Autodesk Inventor part; units mm, degrees
(part 5 of 5)
  arc A545 (140.0996, 136.9129) -> (139.9695, 135.8932) centre (152.2699, 134.8417) ccw projected
  arc A546 (140.8649, 137.1046) -> (140.0996, 136.9129) centre (148.5, 105) ccw projected
  arc A547 (141.4603, 136.2666) -> (140.8649, 137.1046) centre (131.108, 129.5409) ccw projected
  arc A548 (141.8604, 135.5943) -> (141.4603, 136.2666) centre (133.1536, 130.8684) ccw projected
  arc A549 (141.9516, 135.4211) -> (141.8604, 135.5943) centre (135.198, 131.976) ccw projected
  arc A550 (141.9516, 135.4211) -> (142.4946, 135.1579) centre (142.397, 135.6483) ccw projected
  arc A551 (142.5073, 135.1604) -> (142.4946, 135.1579) centre (148.5, 105) ccw projected
  arc A552 (142.5073, 135.1604) -> (142.9083, 135.6114) centre (142.4099, 135.6508) ccw projected
  arc A553 (142.9263, 135.8063) -> (142.9083, 135.6114) centre (150.4662, 135.013) ccw projected
  arc A554 (143.0386, 136.5805) -> (142.9263, 135.8063) centre (152.7789, 134.7721) ccw projected
  arc A555 (143.2681, 137.5826) -> (143.0386, 136.5805) centre (155.1767, 134.3285) ccw projected
  arc A556 (144.0484, 137.6984) -> (143.2681, 137.5826) centre (148.5, 105) ccw projected
  arc A557 (144.5589, 136.8061) -> (144.0484, 137.6984) centre (133.5972, 131.1274) ccw projected
  arc A558 (144.8911, 136.0978) -> (144.5589, 136.8061) centre (135.763, 132.248) ccw projected
  arc A559 (144.9649, 135.9164) -> (144.8911, 136.0978) centre (137.9061, 133.1499) ccw projected
  arc A560 (144.9649, 135.9164) -> (145.4796, 135.6013) centre (145.4304, 136.0989) ccw projected
  arc A561 (145.4924, 135.6026) -> (145.4796, 135.6013) centre (148.5, 105) ccw projected
  arc A562 (145.4924, 135.6026) -> (145.9357, 136.012) centre (145.4435, 136.1002) ccw projected
  arc A563 (145.9727, 136.2043) -> (145.9357, 136.012) centre (153.3985, 134.6758) ccw projected
  arc A564 (146.1603, 136.9638) -> (145.9727, 136.2043) centre (155.6764, 134.2093) ccw projected
  arc A565 (146.4869, 137.9385) -> (146.1603, 136.9638) centre (158.0193, 133.5328) ccw projected
  arc A566 (147.2749, 137.9773) -> (146.4869, 137.9385) centre (148.5, 105) ccw projected
  arc A567 (147.6954, 137.0392) -> (147.2749, 137.9773) centre (136.2299, 132.4624) ccw projected
  arc A568 (147.9566, 136.3017) -> (147.6954, 137.0392) centre (138.4951, 133.3653) ccw projected
  arc A569 (148.0123, 136.1141) -> (147.9566, 136.3017) centre (140.7163, 134.0527) ccw projected
  arc A570 (148.0123, 136.1141) -> (148.4935, 135.75) centre (148.4934, 136.25) ccw projected
  arc A571 (148.5065, 135.75) -> (148.4935, 135.75) centre (148.5, 105) ccw projected
  arc A572 (148.5065, 135.75) -> (148.9877, 136.1141) centre (148.5066, 136.25) ccw projected
  arc A573 (149.0434, 136.3017) -> (148.9877, 136.1141) centre (156.2837, 134.0527) ccw projected
  arc A574 (149.3046, 137.0392) -> (149.0434, 136.3017) centre (158.5049, 133.3653) ccw projected
  arc A575 (149.7251, 137.9773) -> (149.3046, 137.0392) centre (160.7701, 132.4624) ccw projected
  arc A576 (150.5131, 137.9385) -> (149.7251, 137.9773) centre (148.5, 105) ccw projected
  arc A577 (150.8397, 136.9638) -> (150.5131, 137.9385) centre (138.9807, 133.5328) ccw projected
  arc A578 (151.0273, 136.2043) -> (150.8397, 136.9638) centre (141.3236, 134.2093) ccw projected
  arc A579 (151.0643, 136.012) -> (151.0273, 136.2043) centre (143.6015, 134.6758) ccw projected
  arc A580 (151.0643, 136.012) -> (151.5076, 135.6026) centre (151.5565, 136.1002) ccw projected
  arc A581 (151.5204, 135.6013) -> (151.5076, 135.6026) centre (148.5, 105) ccw projected
  arc A582 (151.5204, 135.6013) -> (152.0351, 135.9164) centre (151.5696, 136.0989) ccw projected
  arc A583 (152.1089, 136.0978) -> (152.0351, 135.9164) centre (159.0939, 133.1499) ccw projected
  arc A584 (152.4411, 136.8061) -> (152.1089, 136.0978) centre (161.237, 132.248) ccw projected
  arc A585 (152.9516, 137.6984) -> (152.4411, 136.8061) centre (163.4028, 131.1274) ccw projected
  arc A586 (153.7319, 137.5826) -> (152.9516, 137.6984) centre (148.5, 105) ccw projected
  arc A587 (153.9614, 136.5805) -> (153.7319, 137.5826) centre (141.8233, 134.3285) ccw projected
  arc A588 (154.0737, 135.8063) -> (153.9614, 136.5805) centre (144.2211, 134.7721) ccw projected
  arc A589 (154.0917, 135.6114) -> (154.0737, 135.8063) centre (146.5338, 135.013) ccw projected
  arc A590 (154.0917, 135.6114) -> (154.4927, 135.1604) centre (154.5901, 135.6508) ccw projected
  arc A591 (154.5054, 135.1579) -> (154.4927, 135.1604) centre (148.5, 105) ccw projected
  arc A592 (154.5054, 135.1579) -> (155.0484, 135.4211) centre (154.603, 135.6483) ccw projected
  arc A593 (155.1396, 135.5943) -> (155.0484, 135.4211) centre (161.802, 131.976) ccw projected
  arc A594 (155.5397, 136.2666) -> (155.1396, 135.5943) centre (163.8464, 130.8684) ccw projected
  arc A595 (156.1351, 137.1046) -> (155.5397, 136.2666) centre (165.892, 129.5409) ccw projected
  arc A596 (156.9004, 136.9129) -> (156.1351, 137.1046) centre (148.5, 105) ccw projected
  arc A597 (157.0305, 135.8932) -> (156.9004, 136.9129) centre (144.7301, 134.8417) ccw projected
  arc A598 (157.0664, 135.1116) -> (157.0305, 135.8932) centre (147.1599, 135.0481) ccw projected
  arc A599 (157.0652, 134.9159) -> (157.0664, 135.1116) centre (149.485, 135.0612) ccw projected
  arc A600 (157.0652, 134.9159) -> (157.4201, 134.4278) centre (157.5651, 134.9063) ccw projected
  arc A601 (157.4324, 134.424) -> (157.4201, 134.4278) centre (148.5, 105) ccw projected
  arc A602 (157.4324, 134.424) -> (157.9987, 134.6327) centre (157.5777, 134.9025) ccw projected
  arc A603 (158.1064, 134.7962) -> (157.9987, 134.6327) centre (164.3821, 130.5422) ccw projected
  arc A604 (158.5704, 135.426) -> (158.1064, 134.7962) centre (166.3081, 129.2396) ccw projected
  arc A605 (159.2452, 136.2016) -> (158.5704, 135.426) centre (168.2137, 127.718) ccw projected
  arc A606 (159.988, 135.9358) -> (159.2452, 136.2016) centre (148.5, 105) ccw projected
  arc A607 (160.0175, 134.9083) -> (159.988, 135.9358) centre (147.6733, 135.0675) ccw projected
  arc A608 (159.9766, 134.127) -> (160.0175, 134.9083) centre (150.1116, 135.0348) ccw projected
  arc A609 (159.9562, 133.9323) -> (159.9766, 134.127) centre (152.4268, 134.8199) ccw projected
  arc A610 (159.9562, 133.9323) -> (160.2616, 133.4118) centre (160.4528, 133.8737) ccw projected
  arc A611 (160.2735, 133.4068) -> (160.2616, 133.4118) centre (148.5, 105) ccw projected
  arc A612 (160.2735, 133.4068) -> (160.8574, 133.559) centre (160.4649, 133.8687) ccw projected
  arc A613 (160.9807, 133.7111) -> (160.8574, 133.559) centre (166.8092, 128.8625) ccw projected
  arc A614 (161.5042, 134.2924) -> (160.9807, 133.7111) centre (168.5982, 127.3774) ccw projected
  arc A615 (162.2517, 134.9982) -> (161.5042, 134.2924) centre (170.3455, 125.6763) ccw projected
  arc A616 (162.9649, 134.6609) -> (162.2517, 134.9982) centre (148.5, 105) ccw projected
  arc A617 (162.8936, 133.6353) -> (162.9649, 134.6609) centre (150.6244, 135.0037) ccw projected
  arc A618 (162.7763, 132.8618) -> (162.8936, 133.6353) centre (153.0478, 134.7322) ccw projected
  arc A619 (162.7369, 132.6701) -> (162.7763, 132.8618) centre (155.3308, 134.2914) ccw projected
  arc A620 (162.7369, 132.6701) -> (162.9898, 132.1221) centre (163.2254, 132.5631) ccw projected
  arc A621 (163.0011, 132.116) -> (162.9898, 132.1221) centre (148.5, 105) ccw projected
  arc A622 (163.0011, 132.116) -> (163.5972, 132.2102) centre (163.2369, 132.5569) ccw projected
  arc A623 (163.7348, 132.3495) -> (163.5972, 132.2102) centre (169.06, 126.953) ccw projected
  arc A624 (164.3128, 132.8768) -> (163.7348, 132.3495) centre (170.6948, 125.2996) ccw projected
  arc A625 (165.1258, 133.5058) -> (164.3128, 132.8768) centre (172.267, 123.4355) ccw projected
  arc A626 (165.8025, 133.1002) -> (165.1258, 133.5058) centre (148.5, 105) ccw projected
  arc A627 (165.631, 132.0866) -> (165.8025, 133.1002) centre (153.555, 134.651) ccw projected
  arc A628 (165.4385, 131.3283) -> (165.631, 132.0866) centre (155.9401, 134.1433) ccw projected
  arc A629 (165.3805, 131.1414) -> (165.4385, 131.3283) centre (158.1689, 133.4809) ccw projected
  arc A630 (165.3805, 131.1414) -> (165.5784, 130.5713) centre (165.8561, 130.9871) ccw projected
  arc A631 (165.5891, 130.5641) -> (165.5784, 130.5713) centre (148.5, 105) ccw projected
  arc A632 (165.5891, 130.5641) -> (166.1916, 130.5994) centre (165.867, 130.9798) ccw projected
  arc A633 (166.3421, 130.7246) -> (166.1916, 130.5994) centre (171.1127, 124.8321) ccw projected
  arc A634 (166.969, 131.1926) -> (166.3421, 130.7246) centre (172.5776, 123.0264) ccw projected
  arc A635 (167.8398, 131.7389) -> (166.969, 131.1926) centre (173.9595, 121.0172) ccw projected
  arc A636 (168.4735, 131.269) -> (167.8398, 131.7389) centre (148.5, 105) ccw projected
  arc A637 (168.2035, 130.2771) -> (168.4735, 131.269) centre (156.437, 134.0128) ccw projected
  arc A638 (167.9376, 129.5413) -> (168.2035, 130.2771) centre (158.7608, 133.2737) ccw projected
  arc A639 (167.8615, 129.3609) -> (167.9376, 129.5413) centre (160.914, 132.396) ccw projected
  arc A640 (156.0659, 98.4213) -> (159.5323, 99.2704) centre (155.9652, 106.332) ccw projected
  arc A641 (159.5323, 99.2704) -> (159.9909, 99.7473) centre (159.0814, 100.163) ccw projected
  arc A642 (159.9909, 99.7473) -> (160.3645, 100.6567) centre (148.5, 105) ccw projected
  arc A643 (160.9554, 101.2503) -> (160.3645, 100.6567) centre (161.3036, 100.3129) ccw projected
  arc A644 (160.9554, 101.2503) -> (160.9554, 108.7497) centre (159.5626, 105) ccw projected
  arc A645 (160.3645, 109.3433) -> (160.9554, 108.7497) centre (161.3036, 109.6871) ccw projected
  arc A646 (160.3645, 109.3433) -> (159.9909, 110.2527) centre (148.5, 105) ccw projected
  arc A647 (159.9909, 110.2527) -> (159.5323, 110.7296) centre (159.0814, 109.837) ccw projected
  arc A648 (159.5323, 110.7296) -> (156.0659, 111.5787) centre (155.9652, 103.668) ccw projected
  arc A649 (155.0787, 112.5659) -> (156.0659, 111.5787) centre (156.0787, 112.5787) ccw projected
  arc A650 (155.0787, 112.5659) -> (154.2296, 116.0323) centre (147.168, 112.4652) ccw projected
  arc A651 (154.2296, 116.0323) -> (153.7527, 116.4909) centre (153.337, 115.5814) ccw projected
  arc A652 (153.7527, 116.4909) -> (152.8433, 116.8645) centre (148.5, 105) ccw projected
  arc A653 (152.2497, 117.4554) -> (152.8433, 116.8645) centre (153.1871, 117.8036) ccw projected
  arc A654 (152.2497, 117.4554) -> (144.7503, 117.4554) centre (148.5, 116.0626) ccw projected
  arc A655 (144.1567, 116.8645) -> (144.7503, 117.4554) centre (143.8129, 117.8036) ccw projected
  arc A656 (144.1567, 116.8645) -> (143.2473, 116.4909) centre (148.5, 105) ccw projected
  arc A657 (143.2473, 116.4909) -> (142.7704, 116.0323) centre (143.663, 115.5814) ccw projected
  arc A658 (142.7704, 116.0323) -> (141.9213, 112.5659) centre (149.832, 112.4652) ccw projected
  arc A659 (140.9341, 111.5787) -> (141.9213, 112.5659) centre (140.9213, 112.5787) ccw projected
  arc A660 (140.9341, 111.5787) -> (137.4677, 110.7296) centre (141.0348, 103.668) ccw projected
  arc A661 (137.4677, 110.7296) -> (137.0091, 110.2527) centre (137.9186, 109.837) ccw projected
  arc A662 (137.0091, 110.2527) -> (136.6355, 109.3433) centre (148.5, 105) ccw projected
  arc A663 (136.0446, 108.7497) -> (136.6355, 109.3433) centre (135.6964, 109.6871) ccw projected
  arc A664 (136.0446, 108.7497) -> (136.0446, 101.2503) centre (137.4374, 105) ccw projected
  arc A665 (136.6355, 100.6567) -> (136.0446, 101.2503) centre (135.6964, 100.3129) ccw projected
  arc A666 (136.6355, 100.6567) -> (137.0091, 99.7473) centre (148.5, 105) ccw projected
  arc A667 (137.0091, 99.7473) -> (137.4677, 99.2704) centre (137.9186, 100.163) ccw projected
  arc A668 (137.4677, 99.2704) -> (140.9341, 98.4213) centre (141.0348, 106.332) ccw projected
  arc A669 (141.9213, 97.4341) -> (140.9341, 98.4213) centre (140.9213, 97.4213) ccw projected
  arc A670 (141.9213, 97.4341) -> (142.7704, 93.9677) centre (149.832, 97.5348) ccw projected
  arc A671 (142.7704, 93.9677) -> (143.2473, 93.5091) centre (143.663, 94.4186) ccw projected
  arc A672 (143.2473, 93.5091) -> (144.1567, 93.1355) centre (148.5, 105) ccw projected
  arc A673 (144.7503, 92.5446) -> (144.1567, 93.1355) centre (143.8129, 92.1964) ccw projected
  arc A674 (144.7503, 92.5446) -> (152.2497, 92.5446) centre (148.5, 93.9374) ccw projected
  arc A675 (152.8433, 93.1355) -> (152.2497, 92.5446) centre (153.1871, 92.1964) ccw projected
  arc A676 (152.8433, 93.1355) -> (153.7527, 93.5091) centre (148.5, 105) ccw projected
  arc A677 (153.7527, 93.5091) -> (154.2296, 93.9677) centre (153.337, 94.4186) ccw projected
  arc A678 (154.2296, 93.9677) -> (155.0787, 97.4341) centre (147.168, 97.5348) ccw projected
  arc A679 (156.0659, 98.4213) -> (155.0787, 97.4341) centre (156.0787, 97.4213) ccw projected
  arc A680 (162.8646, 98.8278) -> (162.8646, 111.1722) centre (159.5626, 105) ccw
  arc A681 (162.7193, 98.5) -> (162.8646, 98.8278) centre (148.5, 105) ccw
  arc A682 (160.8849, 96.5927) -> (162.7193, 98.5) centre (159.0814, 100.163) ccw
  arc A683 (157.9055, 95.5945) -> (160.8849, 96.5927) centre (155.9652, 106.332) ccw
  arc A684 (156.9073, 92.6151) -> (157.9055, 95.5945) centre (147.168, 97.5348) ccw
  arc A685 (155, 90.7807) -> (156.9073, 92.6151) centre (153.337, 94.4186) ccw
  arc A686 (154.6722, 90.6354) -> (155, 90.7807) centre (148.5, 105) ccw
  arc A687 (142.3278, 90.6354) -> (154.6722, 90.6354) centre (148.5, 93.9374) ccw
  arc A688 (142, 90.7807) -> (142.3278, 90.6354) centre (148.5, 105) ccw
  arc A689 (140.0927, 92.6151) -> (142, 90.7807) centre (143.663, 94.4186) ccw
  arc A690 (139.0945, 95.5945) -> (140.0927, 92.6151) centre (149.832, 97.5348) ccw
  arc A691 (136.1151, 96.5927) -> (139.0945, 95.5945) centre (141.0348, 106.332) ccw
  arc A692 (134.2807, 98.5) -> (136.1151, 96.5927) centre (137.9186, 100.163) ccw
  arc A693 (134.1354, 98.8278) -> (134.2807, 98.5) centre (148.5, 105) ccw
  arc A694 (134.1354, 111.1722) -> (134.1354, 98.8278) centre (137.4374, 105) ccw
  arc A695 (134.2807, 111.5) -> (134.1354, 111.1722) centre (148.5, 105) ccw
  arc A696 (136.1151, 113.4073) -> (134.2807, 111.5) centre (137.9186, 109.837) ccw
  arc A697 (139.0945, 114.4055) -> (136.1151, 113.4073) centre (141.0348, 103.668) ccw
  arc A698 (140.0927, 117.3849) -> (139.0945, 114.4055) centre (149.832, 112.4652) ccw
  arc A699 (142, 119.2193) -> (140.0927, 117.3849) centre (143.663, 115.5814) ccw
  arc A700 (142.3278, 119.3646) -> (142, 119.2193) centre (148.5, 105) ccw
  arc A701 (154.6722, 119.3646) -> (142.3278, 119.3646) centre (148.5, 116.0626) ccw
  arc A702 (155, 119.2193) -> (154.6722, 119.3646) centre (148.5, 105) ccw
  arc A703 (156.9073, 117.3849) -> (155, 119.2193) centre (153.337, 115.5814) ccw
  arc A704 (157.9055, 114.4055) -> (156.9073, 117.3849) centre (147.168, 112.4652) ccw
  arc A705 (160.8849, 113.4073) -> (157.9055, 114.4055) centre (155.9652, 103.668) ccw
  arc A706 (162.7193, 111.5) -> (160.8849, 113.4073) centre (159.0814, 109.837) ccw
  arc A707 (162.8646, 111.1722) -> (162.7193, 111.5) centre (148.5, 105) ccw
  line L0 (107.811, 105) -> (196.2667, 105) construction
  line L1 (107.811, 102.5) -> (196.2667, 102.5)
  line L2 (196.2667, 107.5) -> (107.811, 107.5)
  arc A708 (107.811, 107.5) -> (107.811, 102.5) centre (107.811, 105) ccw
  arc A709 (196.2667, 102.5) -> (196.2667, 107.5) centre (196.2667, 105) ccw
  line L3 (148.5, 148.8847) -> (148.5, 59.5026) construction
  line L4 (146, 148.8847) -> (146, 59.5026)
  line L5 (151, 59.5026) -> (151, 148.8847)
  arc A710 (151, 148.8847) -> (146, 148.8847) centre (148.5, 148.8847) ccw
  arc A711 (146, 59.5026) -> (151, 59.5026) centre (148.5, 59.5026) ccw
  arc A712 (168.6156, 81.2579) -> (168.0126, 81.234) centre (168.3299, 80.8476) ccw projected
  circle A713 centre (148.5, 105) radius 30.75
  circle A714 centre (148.5, 105) radius 25.75
  point P0 (0, 0)
  point P1 (152.0389, 105)
  point P2 (148.5, 104.1937)
  point P3 (130.8991, 102.5)
  point P4 (122.8716, 102.5)
  point P5 (146, 79.3716)
  point P6 (146, 87.3991)
  point P7 (151, 87.3991)
  point P8 (151, 79.3716)
  point P9 (174.1284, 102.5)
  point P10 (166.1009, 102.5)
  point P11 (166.1009, 107.5)
  point P12 (174.1284, 107.5)
  point P13 (151, 130.6284)
  point P14 (151, 122.6009)
  point P15 (146, 122.6009)
  point P16 (146, 130.6284)
  point P17 (122.8716, 107.5)
  point P18 (130.8991, 107.5)
  dimension "d19" = 3
  dimension "d20" = 5
  dimension "d21" = 5
  dimension "d22" = 5
  constraints: 64 point on circle, 33 centre point, 16 end point, 8 tangent, 2 midpoint, 2 parallel, 2 point on line, 1 coincident, 1 horizontal, 1 perpendicular, 30 other
  measures "d19" radial gap between concentric circles of A680 A644
  measures "d20" diameter of A709
  measures "d21" diameter of A711
extrude "押し出し5" cut sketch "スケッチ5" against normal blind 10 contours A714 L2 A680 A707 A706 A705 A704 A703 A702 A701 L5 | L4 A701 A700 A699 A698 A697 A696 A695 A694 L2 A714 | L1 A714 L5 A687 A686 A685 A684 A683 A682 A681 A680 | L1 A694 A693 A692 A691 A690 A689 A688 A687 L4 A714
fillet "フィレット2" radius 1 20 edges at (122.8716, 102.5, -2.5) (122.8716, 107.5, -2.5) (146, 130.6284, -2.5) (151, 130.6284, -2.5) (174.1284, 107.5, -2.5) (174.1284, 102.5, -2.5) (151, 79.3716, -2.5) (146, 79.3716, -2.5) (134.1354, 98.8278, -2.5) (142.3278, 90.6354, -2.5) (139.0945, 95.5945, -2.5) (154.6722, 90.6354, -2.5) (157.9055, 95.5945, -2.5) (162.8646, 98.8278, -2.5) (162.8646, 111.1722, -2.5) (157.9055, 114.4055, -2.5) (154.6722, 119.3646, -2.5) (142.3278, 119.3646, -2.5) (139.0945, 114.4055, -2.5) (134.1354, 111.1722, -2.5)
fillet "フィレット3" radius 8 8 edges at (130.8991, 102.5, -2.5) (130.8991, 107.5, -2.5) (146, 122.6009, -2.5) (151, 122.6009, -2.5) (166.1009, 107.5, -2.5) (166.1009, 102.5, -2.5) (151, 87.3991, -2.5) (146, 87.3991, -2.5)
